Autodesk Fusion 360 part; units mm, degrees
note: some values were not read from the file. Chosen so that the rebuilt part matches the saved one: a direction; which face or edge a step refers to. Set by a fixed rule: which sketch regions a step uses.
(part 2 of 2)
sketch "Sketch1" plane through (0, 0, 0) normal (0, 0, 1) x (1, 0, 0)
  line L0 (-43.892, 23.418) -> (-3.892, 23.418)
  line L1 (-3.892, 23.418) -> (-3.892, 3.418)
  line L2 (-3.892, 3.418) -> (-43.892, 3.418)
  line L3 (-43.892, 3.418) -> (-43.892, 23.418)
  line L4 (-3.892, 23.418) -> (0.788, 23.418)
  line L5 (3.328, 20.878) -> (3.328, 5.958)
  line L6 (0.788, 3.418) -> (-3.892, 3.418)
  line L7 (-3.892, 3.418) -> (-3.892, 23.418)
  line L8 (-43.892, 23.418) -> (-48.572, 23.418)
  line L9 (-51.112, 20.878) -> (-51.112, 5.958)
  line L10 (-48.572, 3.418) -> (-43.892, 3.418)
  line L11 (-43.892, 3.418) -> (-43.892, 23.418)
  arc A0 (-48.572, 23.418) -> (-51.112, 20.878) centre (-48.572, 20.878) ccw
  arc A1 (-51.112, 5.958) -> (-48.572, 3.418) centre (-48.572, 5.958) ccw
  arc A2 (3.328, 20.878) -> (0.788, 23.418) centre (0.788, 20.878) ccw
  arc A3 (0.788, 3.418) -> (3.328, 5.958) centre (0.788, 5.958) ccw
  line L12 (-47.5817, 23.418) -> (-47.5817, 18.318)
  line L13 (-51.112, 18.318) -> (-48.192, 18.318)
  circle A4 centre (-48.192, 18.318) radius 1.5
  circle A5 centre (-48.192, 8.518) radius 1.5
  line L14 (-47.008, 3.418) -> (-47.008, 8.518)
  line L15 (3.328, 18.8685) -> (0.408, 18.8685)
  circle A6 centre (0.408, 18.318) radius 1.5
  line L16 (-1.3612, 3.418) -> (-1.3612, 8.518)
  circle A7 centre (0.408, 8.518) radius 1.5
  point P0 (3.328, 23.418)
  point P1 (-51.112, 23.418)
  dimension "d1" = 40
  dimension "d2" = 20
  dimension "d3" = 7.22
  dimension "d4" = 20
  dimension "d5" = 7.22
  dimension "d6" = 20
  dimension "d7" = 2.54
  dimension "d8" = 2.54
  dimension "d9" = 5.1
  dimension "d10" = 2.92
  dimension "d11" = 3
  dimension "d13" = 3
  dimension "d14" = 5.1
  dimension "d15" = 2.92
  dimension "d16" = 3
  dimension "d17" = 5.1
  dimension "d18" = 3
  constraint horizontal L0
  constraint vertical L1
  constraint horizontal L2
  constraint vertical L3
  constraint horizontal L4
  constraint vertical L5
  constraint horizontal L6
  constraint vertical L7
  constraint horizontal L8
  constraint vertical L9
  constraint horizontal L10
  constraint vertical L11
  constraint coincident P1 L8
  constraint coincident P1 L9
  constraint tangent L8 A0
  constraint tangent L9 A0
  constraint tangent L9 A1
  constraint tangent L10 A1
  constraint coincident P0 L4
  constraint coincident P0 L5
  constraint tangent L4 A2
  constraint tangent L5 A2
  constraint equal A1 A2
  constraint tangent L5 A3
  constraint tangent L6 A3
  constraint equal A1 A3
  constraint coincident L8 L12.start
  constraint perpendicular L8 L12
  constraint coincident L9 L13.start
  constraint perpendicular L12 L13
  constraint coincident L13.end A4.centre
  constraint coincident L10 L14.start
  constraint perpendicular L10 L14
  constraint coincident L5 L15.start
  constraint perpendicular L5 L15
  constraint coincident L6 L16.start
  constraint perpendicular L6 L16
  measures "d1" distance of L0.start L0.end
  measures "d2" distance of L0.start L2.end
  measures "d3" distance of L0.end P0
  measures "d4" distance of L0.end L1.end
  measures "d5" distance of L0.start P1
  measures "d6" distance of L0.start L2.end
  measures "d7" radius of A0
  measures "d8" radius of A1
  measures "d9" distance of L12.start L12.end
  measures "d10" distance of L13.start L13.end
  measures "d11" diameter of A4
  measures "d13" diameter of A5
  measures "d14" distance of L14.start L14.end
  measures "d15" distance of L15.start L15.end
  measures "d16" diameter of A6
  measures "d17" distance of L16.start L16.end
  measures "d18" diameter of A7
extrude "Extrude1" add sketch "Sketch1" along normal blind 3.175 contours L0 L1 L2 L3 L7 L11 | L3 L8 L9 L10 L11 A1 L12 L13 A4 | L1 L4 L5 L6 L7 A2 A3 | L8 L9 A0 L12 L13 A4 makes body 1
sketch "Sketch2" plane through (0, 0, 0) normal (0, 0, -1) x (1, 0, 0)
  circle A0 centre (0.408, -18.318) radius 1.5
  circle A1 centre (-48.192, -18.318) radius 1.5
  circle A2 centre (0.408, -8.518) radius 1.5
  circle A3 centre (-48.192, -8.518) radius 1.5
  line L0 (0.788, -3.418) -> (-48.572, -3.418)
  arc A4 (-48.572, -3.418) -> (-51.112, -5.958) centre (-48.572, -5.958) ccw
  line L1 (-51.112, -5.958) -> (-51.112, -20.878)
  arc A5 (-51.112, -20.878) -> (-48.572, -23.418) centre (-48.572, -20.878) ccw
  line L2 (-48.572, -23.418) -> (0.788, -23.418)
  arc A6 (0.788, -23.418) -> (3.328, -20.878) centre (0.788, -20.878) ccw
  line L3 (3.328, -20.878) -> (3.328, -5.958)
  arc A7 (3.328, -5.958) -> (0.788, -3.418) centre (0.788, -5.958) ccw
  line L4 (-51.112, -13.418) -> (-43.892, -13.418)
  line L5 (-43.892, -5.958) -> (-43.892, -20.878)
  line L6 (-41.352, -3.418) -> (-6.432, -3.418)
  line L7 (-3.892, -5.958) -> (-3.892, -20.878)
  line L8 (-6.432, -23.418) -> (-41.352, -23.418)
  arc A8 (-41.352, -3.418) -> (-43.892, -5.958) centre (-41.352, -5.958) ccw
  arc A9 (-43.892, -20.878) -> (-41.352, -23.418) centre (-41.352, -20.878) ccw
  arc A10 (-3.892, -5.958) -> (-6.432, -3.418) centre (-6.432, -5.958) ccw
  arc A11 (-6.432, -23.418) -> (-3.892, -20.878) centre (-6.432, -20.878) ccw
  point P0 (-43.892, -3.418)
  point P1 (-3.892, -3.418)
  dimension "d21" = 7.22
  dimension "d22" = 40
  dimension "d23" = 2.54
  constraint midpoint L1 L4.start
  constraint perpendicular L1 L4
  constraint coincident L0 P0
  constraint perpendicular L2 L5
  constraint coincident L0 P1
  constraint perpendicular L2 L7
  constraint coincident P0 L5
  constraint coincident P0 L6
  constraint tangent L5 A8
  constraint tangent L6 A8
  constraint tangent L5 A9
  constraint tangent L8 A9
  constraint equal A8 A9
  constraint coincident P1 L6
  constraint coincident P1 L7
  constraint tangent L6 A10
  constraint tangent L7 A10
  constraint equal A8 A10
  constraint tangent L7 A11
  constraint tangent L8 A11
  constraint equal A8 A11
  measures "d21" distance of L4.start L4.end
  measures "d22" distance of P0 P1
  measures "d23" radius of A8
extrude "Extrude2" add sketch "Sketch2" along normal blind 27.65 contours L0 L2 L5 L6 L7 L8 A8 A9 A10 A11 bodies 1
sketch "Sketch3" plane through (0, 0, 3.175) normal (0, 0, 1) x (-1, 0, 0)
  circle A0 centre (-0.408, -18.318) radius 1.5
  circle A1 centre (48.192, -18.318) radius 1.5
  circle A2 centre (-0.408, -8.518) radius 1.5
  circle A3 centre (48.192, -8.518) radius 1.5
  line L0 (48.572, -3.418) -> (-0.788, -3.418)
  arc A4 (-0.788, -3.418) -> (-3.328, -5.958) centre (-0.788, -5.958) ccw
  line L1 (-3.328, -5.958) -> (-3.328, -20.878)
  arc A5 (-3.328, -20.878) -> (-0.788, -23.418) centre (-0.788, -20.878) ccw
  line L2 (-0.788, -23.418) -> (48.572, -23.418)
  arc A6 (48.572, -23.418) -> (51.112, -20.878) centre (48.572, -20.878) ccw
  line L3 (51.112, -20.878) -> (51.112, -5.958)
  arc A7 (51.112, -5.958) -> (48.572, -3.418) centre (48.572, -5.958) ccw
  line L4 (51.112, -13.418) -> (43.892, -13.418)
  line L5 (43.892, -13.418) -> (43.892, -20.878)
  line L6 (41.352, -23.418) -> (6.432, -23.418)
  line L7 (3.892, -20.878) -> (3.892, -5.958)
  line L8 (43.892, -13.418) -> (43.892, -5.958)
  line L9 (41.352, -3.418) -> (6.432, -3.418)
  arc A8 (41.352, -23.418) -> (43.892, -20.878) centre (41.352, -20.878) ccw
  arc A9 (43.892, -5.958) -> (41.352, -3.418) centre (41.352, -5.958) ccw
  arc A10 (6.432, -3.418) -> (3.892, -5.958) centre (6.432, -5.958) ccw
  arc A11 (3.892, -20.878) -> (6.432, -23.418) centre (6.432, -20.878) ccw
  point P0 (43.892, -23.418)
  point P1 (3.892, -23.418)
  dimension "d26" = 7.22
  dimension "d27" = 40
  dimension "d28" = 2.54
  constraint midpoint L3 L4.start
  constraint perpendicular L3 L4
  constraint coincident L2 P0
  constraint perpendicular L2 L5
  constraint perpendicular L5 L6
  constraint perpendicular L0 L7
  constraint perpendicular L0 L8
  constraint coincident P0 L5
  constraint coincident P0 L6
  constraint tangent L5 A8
  constraint tangent L6 A8
  constraint tangent L8 A9
  constraint tangent L9 A9
  constraint equal A8 A9
  constraint tangent L7 A10
  constraint tangent L9 A10
  constraint equal A8 A10
  constraint coincident P1 L6
  constraint coincident P1 L7
  constraint tangent L6 A11
  constraint tangent L7 A11
  constraint equal A8 A11
  measures "d26" distance of L4.start L4.end
  measures "d27" distance of P0 P1
  measures "d28" radius of A8
extrude "Extrude3" add sketch "Sketch3" along normal blind 9.525 contours L0 L2 L5 L6 L7 L8 L9 A8 A9 A10 A11 bodies 1
sketch "Sketch4" plane through (0, 0, 12.7) normal (0, 0, 1) x (-1, 0, 0)
  line L0 (43.892, -20.878) -> (43.892, -5.958)
  arc A0 (43.892, -5.958) -> (41.352, -3.418) centre (41.352, -5.958) ccw
  line L1 (41.352, -3.418) -> (6.432, -3.418)
  arc A1 (6.432, -3.418) -> (3.892, -5.958) centre (6.432, -5.958) ccw
  line L2 (3.892, -5.958) -> (3.892, -20.878)
  arc A2 (3.892, -20.878) -> (6.432, -23.418) centre (6.432, -20.878) ccw
  line L3 (6.432, -23.418) -> (41.352, -23.418)
  arc A3 (41.352, -23.418) -> (43.892, -20.878) centre (41.352, -20.878) ccw
  line L4 (43.892, -13.418) -> (13.742, -13.418)
  circle A4 centre (13.742, -13.418) radius 5
  circle A5 centre (13.742, -13.418) radius 2.5
  dimension "d31" = 30.15
  dimension "d32" = 10
  dimension "d33" = 5
  constraint midpoint L0 L4.start
  constraint perpendicular L0 L4
  constraint coincident L4.end A4.centre
  constraint concentric A4 A5
  measures "d31" distance of L4.start L4.end
  measures "d32" diameter of A4
  measures "d33" diameter of A5
extrude "Extrude4" add sketch "Sketch4" along normal blind 6.35 contours A4 bodies 1
sketch "Sketch5" plane through (0, 0, 19.05) normal (0, 0, 1) x (-1, 0, 0)
  circle A0 centre (13.742, -13.418) radius 2.5
  circle A1 centre (13.742, -13.418) radius 5
sketch "Sketch6" plane through (0, 0, 19.05) normal (0, 0, 1) x (-1, 0, 0)
sketch "Sketch7" plane through (0, 0, 19.05) normal (0, 0, 1) x (-1, 0, 0)
sketch "Sketch8" plane through (0, 0, 12.7) normal (0, 0, 1) x (-1, 0, 0)
  line L0 (43.892, -20.878) -> (43.892, -5.958)
  arc A0 (43.892, -5.958) -> (41.352, -3.418) centre (41.352, -5.958) ccw
  line L1 (41.352, -3.418) -> (6.432, -3.418)
  arc A1 (6.432, -3.418) -> (3.892, -5.958) centre (6.432, -5.958) ccw
  line L2 (3.892, -5.958) -> (3.892, -20.878)
  arc A2 (3.892, -20.878) -> (6.432, -23.418) centre (6.432, -20.878) ccw
  line L3 (6.432, -23.418) -> (41.352, -23.418)
  arc A3 (41.352, -23.418) -> (43.892, -20.878) centre (41.352, -20.878) ccw
  circle A4 centre (13.742, -13.418) radius 5
  line L4 (13.742, -13.418) -> (13.742, -29.928)
  line L5 (13.742, -13.418) -> (-2.768, -13.418)
  line L6 (13.742, -13.418) -> (30.252, -13.418) construction
  line L7 (13.742, -13.418) -> (30.252, -13.418)
  line L8 (13.742, -13.418) -> (30.252, -13.418) construction
  line L9 (10.567, -13.418) -> (10.567, -29.928)
  arc A5 (10.567, -29.928) -> (16.917, -29.928) centre (13.742, -29.928) ccw
  line L10 (16.917, -29.928) -> (16.917, -13.418)
  arc A6 (16.917, -13.418) -> (10.567, -13.418) centre (13.742, -13.418) ccw
  line L11 (13.742, -13.418) -> (13.742, -29.928) construction
  line L12 (13.742, -10.243) -> (-2.768, -10.243)
  arc A7 (-2.768, -10.243) -> (-2.768, -16.593) centre (-2.768, -13.418) ccw
  line L13 (-2.768, -16.593) -> (13.742, -16.593)
  arc A8 (13.742, -16.593) -> (13.742, -10.243) centre (13.742, -13.418) ccw
  line L14 (13.742, -13.418) -> (-2.768, -13.418) construction
  line L15 (13.742, -16.593) -> (30.252, -16.593)
  arc A9 (30.252, -16.593) -> (30.252, -10.243) centre (30.252, -13.418) ccw
  line L16 (30.252, -10.243) -> (13.742, -10.243)
  arc A10 (13.742, -10.243) -> (13.742, -16.593) centre (13.742, -13.418) ccw
  line L17 (13.742, -13.418) -> (30.252, -13.418) construction
  circle A11 centre (13.742, -29.928) radius 0.9525
  circle A12 centre (-2.768, -13.418) radius 0.9525
  circle A13 centre (30.252, -13.418) radius 0.9525
  line L18 (13.742, -13.418) -> (13.742, 3.092)
  line L19 (16.917, -13.418) -> (16.917, 3.092)
  arc A14 (16.917, 3.092) -> (10.567, 3.092) centre (13.742, 3.092) ccw
  line L20 (10.567, 3.092) -> (10.567, -13.418)
  arc A15 (10.567, -13.418) -> (16.917, -13.418) centre (13.742, -13.418) ccw
  line L21 (13.742, -13.418) -> (13.742, 3.092) construction
  circle A16 centre (13.742, 3.092) radius 0.9525
  dimension "d36" = 16.51
  dimension "d38" = 16.51
  dimension "d40" = 16.51
  dimension "d41" = 6.35
  dimension "d42" = 6.35
  dimension "d43" = 6.35
  dimension "d44" = 1.905
  dimension "d45" = 1.905
  dimension "d46" = 1.905
  dimension "d49" = 16.51
  dimension "d50" = 6.35
  dimension "d51" = 1.905
  constraint coincident A4.centre L4.start
  constraint perpendicular L3 L4
  constraint horizontal L6
  constraint horizontal L8
  constraint tangent L9 A5
  constraint tangent A5 L10
  constraint parallel L9 L10
  constraint tangent L10 A6
  constraint tangent L9 A6
  constraint coincident L4.end A5.centre
  constraint perpendicular L6 L11
  constraint tangent L12 A7
  constraint tangent A7 L13
  constraint parallel L12 L13
  constraint tangent L13 A8
  constraint tangent L12 A8
  constraint coincident L5.end A7.centre
  constraint parallel L5 L14
  constraint tangent L15 A9
  constraint tangent A9 L16
  constraint parallel L15 L16
  constraint tangent L16 A10
  constraint tangent L15 A10
  constraint coincident L6.end L7.end
  constraint parallel L7 L17
  constraint concentric A7 A12
  constraint concentric A9 A13
  constraint perpendicular L12 L18
  constraint tangent L19 A14
  constraint tangent A14 L20
  constraint parallel L19 L20
  constraint tangent L20 A15
  constraint tangent L19 A15
  constraint coincident L18.end A14.centre
  constraint perpendicular L17 L21
  constraint concentric A14 A16
  measures "d36" distance of A4.centre L4.end
  measures "d38" distance of A4.centre L5.end
  measures "d40" distance of A4.centre L6.end
  measures "d41" diameter of A5
  measures "d42" diameter of A7
  measures "d43" diameter of A9
  measures "d44" diameter of A11
  measures "d45" diameter of A12
  measures "d46" diameter of A13
  measures "d49" distance of A4.centre L18.end
  measures "d50" diameter of A14
  measures "d51" diameter of A16
extrude "Extrude5" add sketch "Sketch8" along normal blind 2.54 separate body contours L3 L9 A5 L10 | L3 A4 L4 L10 | L1 A4 L18 L19 | L1 L19 A14 L20 | L3 A4 L4 L9 | A4 L10 L15 | A4 L4 L10 L15 | L1 A4 L18 L20 | A4 L16 L18 L19 | A4 L16 L19 | A4 L4 L9 L13 | A4 L7 L10 L15 | A4 L15 A9 L16 | L10 A8 L15 A15 | A4 L12 L18 L20 | A4 L7 L16 L19 | A6 A8 L16 L19 | A4 L9 L13 | L9 L13 A10 A15 | A4 L12 L20 | A6 L12 A10 L20 | L2 A4 L5 L13 | A4 L5 L9 L13 | A4 L5 L12 L20 | L2 A4 L5 L12 | L2 L12 A7 L13 makes body 2
move_body "Move1" bodies 2 to x (1, 0, 0) y (0, 1, 0) z (0, 0, 1) at (0, 0, 5.08)
move_body "Move2" bodies 2 to x (1, 0, 0) y (0, 1, 0) z (0, 0, 1) at (0, 0, 1.27)
move_body "Move3" bodies 2 to x (1, 0, 0) y (0, 1, 0) z (0, 0, 1) at (0, 0, 0.635)
move_body "Move4" bodies 2 to x (1, 0, 0) y (0, 1, 0) z (0, 0, 1) at (0, 0, -0.635)
combine "Combine1" operation add target body 1 tool bodies 2
equation "d19 = ( 1 / 8 ) * 1 in"
named bodies: "Servo"
